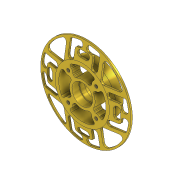
# Autodesk Inventor part: base
Saved by Autodesk Inventor 2020 (Build 240168000, 168)
## iProperties
Created: 2020-05-19
Part Number: base
Material: Generic
Document SubType Name: Modeling
Designer: Kostic
Density: 1 g/cm^3
Appearance: Aluminum - Polished
Author: Kostic
Autodesk Inventor part; units mm, degrees
ref_plane "YZ Plane" through (0, 0, 0) normal (1, 0, 0) x (0, 1, 0)
ref_plane "XZ Plane" through (0, 0, 0) normal (0, 1, 0) x (-1, 0, 0)
ref_plane "XY Plane" through (0, 0, 0) normal (0, 0, 1) x (1, 0, 0)
sketch "Sketch1" plane through (0, 0, 0) normal (0, 0, 1) x (1, 0, 0)
  circle A0 centre (0, 0) radius 24
  circle A1 centre (0, 0) radius 27.5
  dimension "d0" = 48
  dimension "d1" = 55
  constraints: 2 centre point, 2 coincident
  measures "d0" diameter of A0
  measures "d1" diameter of A1
extrude "Extrusion1" add sketch "Sketch1" along normal blind 2
sketch "Sketch2" plane through (0, 0, 0) normal (0, 0, -1) x (-1, 0, 0)
  circle A0 centre (0, 0) radius 24
  circle A1 centre (0, 0) radius 26
  dimension "d4" = 52
  constraints: 2 centre point, 2 coincident
  measures "d4" diameter of A1
extrude "Extrusion2" add sketch "Sketch2" along normal blind 13.6
sketch "Sketch3" plane through (0, 0, 0) normal (1, 0, 0) x (0, 1, 0)
  line L0 (45.8, -1.5) -> (45.8, -3.1)
  line L1 (27.5, 2) -> (-27.5, 2) projected
  line L2 (-24, 2) -> (24, 2) projected
  line L3 (0, 2) -> (0, -26.5)
  line L4 (45.8, -1.5) -> (27.5, 2)
  line L5 (27.5, 0) -> (-27.5, 0) projected
  line L6 (45.8, -3.1) -> (27.5, 0)
  line L7 (27.5, 0) -> (27.5, 2)
  line L8 (27.5, 0) -> (27.5, 2) projected
  point P0 (0, 0)
  dimension "d7" = 1.6
  dimension "d8" = 45.8
  dimension "d9" = 3.5
  dimension "d10" = 28.5
  dimension "d11" = 25
  constraints: 10 end point, 2 vertical, 1 collinear, 1 midpoint
  measures "d7" distance of L0.start L0.end
  measures "d8" distance from line of point (0, 0) L0
  measures "d9" distance from line of L0.start L1
  measures "d10" distance of L3.start L3.end
  measures "d11" vertical distance of L0.start L3.end
revolve "Revolution1" add sketch "Sketch3" angle 360 about axis through (0, 0, 2) along (0, 0, -1) contours L0 L6 L7 L4
sketch "Sketch4" plane through (0, 0, 2) normal (0, 0, 1) x (1, 0, 0)
  line L0 (0, 64.12) -> (0, -64.12) projected
  circle A0 centre (0, 0) radius 24 projected
  line L1 (15, 28.0401) -> (9, 28.0401)
  arc A1 (9, 28.0401) -> (15, 28.0401) centre (12, 28.0401) ccw
  circle A2 centre (0, 0) radius 27.5 projected
  circle A3 centre (0, 0) radius 44 construction
  arc A4 (13.619, 41.8392) -> (5.3659, 43.6716) centre (0, 0) ccw
  circle A5 centre (5, 40.694) radius 3
  arc A6 (7.3889, 37.2748) -> (4.6154, 37.7187) centre (0, 0) ccw
  line L2 (15, 39.9375) -> (15, 28.0401)
  line L3 (9, 28.0401) -> (9, 35.313)
  arc A7 (15, 39.9375) -> (13.619, 41.8392) centre (13, 39.9375) ccw
  arc A8 (9, 35.313) -> (7.3889, 37.2748) centre (7, 35.313) ccw
  line L4 (0, 37) -> (3, 37)
  line L5 (6, 34) -> (6, 34)
  line L6 (3, 31) -> (0, 31)
  line L7 (0, 31) -> (0, 37)
  arc A9 (6, 34) -> (3, 37) centre (3, 34) ccw
  arc A10 (3, 31) -> (6, 34) centre (3, 34) ccw
  line L8 (0, 0) -> (39.4119, 39.4119) construction
  line L9 (0, 0) -> (55.7369, 0) construction
  circle A11 centre (21.5668, 21.5668) radius 3
  circle A12 centre (0, 0) radius 27.5 projected
  line L10 (18.5668, 21.5668) -> (18.5668, 34.8694)
  line L11 (21.5668, 18.5668) -> (34.8694, 18.5668)
  arc A13 (37.4208, 23.1448) -> (23.1448, 37.4208) centre (0, 0) ccw
  arc A14 (23.1448, 37.4208) -> (18.5668, 34.8694) centre (21.5668, 34.8694) ccw
  arc A15 (34.8694, 18.5668) -> (37.4208, 23.1448) centre (34.8694, 21.5668) ccw
  line L12 (19.4454, 19.4454) -> (31.1127, 31.1127)
  point P0 (15, 41.3642)
  point P1 (9, 36.9189)
  point P2 (6, 31)
  point P3 (6, 37)
  point P4 (18.5668, 39.8908)
  point P5 (39.8908, 18.5668)
  point P6 (0, 31)
  dimension "d17" = 6
  dimension "d18" = 3
  dimension "d19" = 88
  dimension "d20" = 44
  dimension "d21" = 6
  dimension "d22" = 5
  dimension "d25" = 15
  dimension "d27" = 2
  dimension "d28" = 2
  dimension "d32" = 38.0001
  dimension "d33" = 6
  dimension "d34" = 6
  dimension "d35" = 6
  dimension "d36" = 31
  dimension "d37" = 3
  dimension "d38" = 45
  dimension "d39" = 6
  dimension "d40" = 44
  dimension "d41" = 3
  constraints: 30 point on circle, 24 end point, 14 tangent, 13 centre point, 10 point on line, 4 coincident, 3 horizontal, 3 parallel, 2 equal radius, 1 equal length, 1 perpendicular, 1 vertical, 3 other
  measures "d17" distance of L1.start L1.end
  measures "d18" radius of A1
  measures "d19" diameter of A3
  measures "d20" radius of A4
  measures "d21" diameter of A5
  measures "d22" distance from line of L0 A5.centre
  measures "d25" distance between parallel lines of L0 L2
  measures "d27" radius of A7
  measures "d28" radius of A8
  measures "d32" radius of A6
  measures "d33" distance between parallel lines of L2 L3
  measures "d34" distance of point (6, 31) L6.end
  measures "d35" distance of point (6, 37) point (6, 31)
  measures "d36" distance from line of point (0, 0) L6
  measures "d37" radius of A9
  measures "d38" angle of L9 L8
  measures "d39" diameter of A11
  measures "d40" radius of A13
  measures "d41" radius of A14
extrude "Extrusion3" cut sketch "Sketch4" against normal blind 10 contours L4 A9 A10 L6 L0 | A1 L1 | A11 L12 | L3 A8 A6 A5 A4 A7 L2 L1 | L10 A14 A13 L12 A11 | A5 picked at (20.6429, 21.1841)
mirror "Mirror1" about plane through (0, 31, 2) normal (1, 0, 0) of "Extrusion3"
pattern_circular "Circular Pattern1" count 4 over 360 about axis through (0, 0, 0) along (0, 0, 1) of "Extrusion3", "Mirror1"
sketch "Sketch5" plane through (0, 0, 2) normal (0, 0, 1) x (1, 0, 0)
  circle A0 centre (0, 0) radius 10.5
  circle A1 centre (0, 0) radius 13
  line L0 (0, 0) -> (45.9095, 45.9095) construction
  line L1 (0, 0) -> (64.9258, 0) construction
  circle A2 centre (14.1421, 14.1421) radius 1.5
  circle A3 centre (14.1421, 14.1421) radius 4.5
  line L2 (6.3374, 9.8729) -> (9.9759, 13.5115)
  line L3 (9.9759, 13.5115) -> (13.5115, 9.9759)
  line L4 (13.5115, 9.9759) -> (9.8729, 6.3374)
  line L5 (9.8729, 6.3374) -> (6.3374, 9.8729)
  line L6 (10.9602, 17.3241) -> (13.4876, 19.8516)
  circle A4 centre (0, 0) radius 24 projected
  line L7 (10.9602, 17.3241) -> (14.5345, 17.3241) construction
  line L8 (17.3241, 10.9602) -> (19.8516, 13.4876)
  line L9 (17.3241, 10.9602) -> (20.8985, 10.9602) construction
  point P0 (9.7286, 13.2642)
  point P1 (7.253, 10.7886)
  point P2 (10.7886, 7.253)
  point P3 (13.2642, 9.7286)
  dimension "d47" = 21
  dimension "d48" = 26
  dimension "d49" = 45
  dimension "d50" = 3
  dimension "d51" = 20
  dimension "d52" = 9
  dimension "d53" = 5
  dimension "d54" = 2.5
  dimension "d55" = 45
  dimension "d56" = 45
  constraints: 20 end point, 4 centre point, 4 point on circle, 3 coincident, 3 equal length, 3 horizontal, 3 parallel, 2 tangent, 1 perpendicular, 1 point on line
  measures "d47" diameter of A0
  measures "d48" diameter of A1
  measures "d49" angle of L1 L0
  measures "d50" diameter of A2
  measures "d51" distance of point (0, 0) A2.centre
  measures "d52" diameter of A3
  measures "d53" distance of L2.end L3.end
  measures "d54" distance between parallel lines of L0 L2
  measures "d55" angle of L7 L6
  measures "d56" angle of L9 L8
extrude "Extrusion4" add sketch "Sketch5" against normal up to surface (15.6 mm away) contours A1 L2 L5 L4 | L4 L5 L2 A1 | A1 L2 A3 L4 | L4 L3 L2 A3 A4 | A3 L2 L3 L4 | A3 A4 L8 | L6 A4 A3 | A2
fillet "Fillet1" radius 2 8 edges at (19.8516, 13.4876, 1) (19.8516, 13.4876, -6.8) (13.4876, 19.8516, 1) (13.4876, 19.8516, -6.8) (13.2642, 9.7286, -5.8) (9.7286, 13.2642, -5.8) (7.253, 10.7886, -5.8) (10.7886, 7.253, -5.8)
sketch "Sketch6" plane through (0, 0, 2) normal (0, 0, 1) x (1, 0, 0)
  arc A0 (14.0489, 9.6431) -> (17.3241, 10.9602) centre (14.1421, 14.1421) ccw projected
  point P0 (0, 0)
  constraints: 1 coincident
hole "Hole1" at (14.1421, 14.1421, 2) direction (0, 0, -1) diameter 3.242 end through all thread size "M4x0.7" class "6H" standard "ISO Metric profile"
pattern_circular "Circular Pattern2" count 4 over 360 about axis through (0, 0, 2) along (0, 0, -1) of "Extrusion4", "Fillet1", "Hole1"
sketch "Sketch7" plane through (0, 0, -13.6) normal (0, 0, -1) x (-1, 0, 0)
  circle A0 centre (0, 0) radius 24
  circle A1 centre (0, 0) radius 13
  constraints: 2 centre point, 2 coincident
extrude "Extrusion5" cut sketch "Sketch7" against normal blind 8
sketch "Sketch8" plane through (0, 0, 0) normal (0, 0, -1) x (-1, 0, 0)
  circle A0 centre (0, 0) radius 26
  circle A1 centre (0, 0) radius 26.5
  dimension "d72" = 53
  constraints: 2 centre point, 2 coincident
  measures "d72" diameter of A1
extrude "Extrusion6" add sketch "Sketch8" along normal blind 5.6
sketch "Sketch9" plane through (0, 0, -13.6) normal (0, 0, -1) x (-1, 0, 0)
  circle A0 centre (0, 0) radius 10.5
  circle A1 centre (0, 0) radius 9.5
  dimension "d75" = 19
  constraints: 2 centre point, 2 coincident
  measures "d75" diameter of A1
extrude "Extrusion7" add sketch "Sketch9" against normal blind 8.6
sketch "Sketch10" plane through (0, 0, -13.6) normal (0, 0, -1) x (-1, 0, 0)
  circle A0 centre (0, 0) radius 9.5
  circle A1 centre (0, 0) radius 9.5 projected
  circle A2 centre (0, 0) radius 10.5
  dimension "d78" = 21
  constraints: 2 centre point, 2 coincident
  measures "d78" diameter of A2
extrude "Extrusion8" cut sketch "Sketch10" against normal blind 4
body "Solid1"
